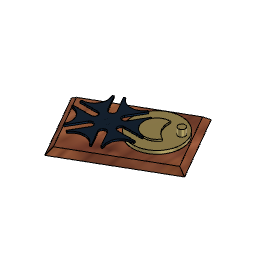
second mechanism v1 (Autodesk Fusion 360 design; units mm, degrees)
Autodesk Fusion 360 part; units mm, degrees
sketch "all" plane through (0, 0, 0) normal (0, 0, 1) x (1, 0, 0) in component "holder"
  circle A0 centre (-15, -0.013468) radius 19
  circle A1 centre (4, 10.956187) radius 7.95
  circle A2 centre (4, -0.013468) radius 2.099973
  line L0 (-15, -0.013468) -> (4, -0.013468) construction
  line L1 (4, -0.013468) -> (4, 10.956187) construction
  circle A3 centre (4, 10.956187) radius 10.969655 construction
  line L2 (4, 10.956187) -> (-5.5, 5.47136) construction
  line L3 (4, 2.086505) -> (-6.969655, 2.086505)
  arc A4 (-6.969655, 2.086505) -> (-6.969655, -2.113441) centre (-6.969655, -0.013468) ccw
  line L4 (-6.969655, -2.113441) -> (4, -2.113441)
  arc A5 (4, -2.113441) -> (4, 2.086505) centre (4, -0.013468) ccw
  line L5 (4, -0.013468) -> (-6.969655, -0.013468) construction
  circle A6 centre (-15, 21.925842) radius 7.95
  line L6 (-9.166198, 5.891028) -> (-3.68137, 15.391028)
  arc A7 (-12.803457, 7.991001) -> (-9.166198, 5.891028) centre (-10.984827, 6.941015) ccw
  line L7 (-7.31863, 17.491001) -> (-12.803457, 7.991001)
  arc A8 (-3.68137, 15.391028) -> (-7.31863, 17.491001) centre (-5.5, 16.441015) ccw
  circle A9 centre (-34, 10.956187) radius 7.95
  line L8 (-17.196543, 7.991001) -> (-22.68137, 17.491001)
  arc A10 (-20.833802, 5.891028) -> (-17.196543, 7.991001) centre (-19.015172, 6.941015) ccw
  line L9 (-26.31863, 15.391028) -> (-20.833802, 5.891028)
  arc A11 (-22.68137, 17.491001) -> (-26.31863, 15.391028) centre (-24.5, 16.441015) ccw
  circle A12 centre (-34, -10.983123) radius 7.95
  line L10 (-23.030345, 2.086505) -> (-34, 2.086505)
  arc A13 (-23.030345, -2.113441) -> (-23.030345, 2.086505) centre (-23.030345, -0.013468) ccw
  line L11 (-34, -2.113441) -> (-23.030345, -2.113441)
  arc A14 (-34, 2.086505) -> (-34, -2.113441) centre (-34, -0.013468) ccw
  circle A15 centre (-15, -21.952778) radius 7.95
  line L12 (-20.833802, -5.917964) -> (-26.31863, -15.417964)
  arc A16 (-17.196543, -8.017937) -> (-20.833802, -5.917964) centre (-19.015172, -6.967951) ccw
  line L13 (-22.68137, -17.517937) -> (-17.196543, -8.017937)
  arc A17 (-26.31863, -15.417964) -> (-22.68137, -17.517937) centre (-24.5, -16.467951) ccw
  circle A18 centre (4, -10.983123) radius 7.95
  line L14 (-12.803457, -8.017937) -> (-7.31863, -17.517937)
  arc A19 (-9.166198, -5.917964) -> (-12.803457, -8.017937) centre (-10.984827, -6.967951) ccw
  line L15 (-3.68137, -15.417964) -> (-9.166198, -5.917964)
  arc A20 (-7.31863, -17.517937) -> (-3.68137, -15.417964) centre (-5.5, -16.467951) ccw
  circle A21 centre (-15, -0.013468) radius 2
  line L16 (14.89621, 17.518771) -> (14.508328, 17.285157)
  line L17 (-34, -10.983123) -> (-45, 8.069436)
  line L18 (-34, -10.983123) -> (-23, -30.035682)
  line L19 (-45, 8.069436) -> (2.631397, 35.569436)
  line L20 (-23, -30.035682) -> (24.631397, -2.535682)
  line L21 (26.363448, -1.535682) -> (24.631397, -2.535682)
  line L22 (4.363448, 36.569436) -> (2.631397, 35.569436)
  circle A22 centre (4, 10.956187) radius 1.5
  circle A23 centre (4, 10.956187) radius 14.790733
  line L23 (30.693575, 0.964318) -> (8.693575, 39.069436)
  line L24 (30.693575, 0.964318) -> (26.363448, -1.535682)
  line L25 (8.693575, 39.069436) -> (4.363448, 36.569436)
  line L26 (4, 10.956187) -> (0.025, 17.841089)
  line L27 (4, 10.956187) -> (7.975, 4.071285)
  line L28 (-0.75, 8.213773) -> (22.60208, 21.696103)
  circle A24 centre (15.672989, 17.69559) radius 11.407497
  dimension "d3" = 38
  dimension "d8" = 360
  dimension "d9" = 4
  dimension "d10" = 15.9
  dimension "d11" = 22
  dimension "d12" = 22
  dimension "d13" = 55
  dimension "d14" = 55
  dimension "d15" = 55
  dimension "d17" = 3
  constraint horizontal L0
  constraint tangent A0 L1
  constraint perpendicular L0 L1
  constraint concentric A1 A3
  constraint tangent L3 A4
  constraint tangent A4 L4
  constraint parallel L3 L4
  constraint tangent L4 A5
  constraint tangent L3 A5
  constraint parallel L0 L5
  constraint equal A2 A5
  constraint equal L2 L5
  constraint concentric A0 A21
  constraint perpendicular L17 L19
  constraint perpendicular L18 L20
  constraint concentric A1 A22
  constraint concentric A3 A23
  constraint perpendicular L2 L26
  constraint perpendicular L2 L27
  constraint perpendicular L23 L28
  measures "d3" diameter of A0
  measures "d9" diameter of A21
  measures "d10" diameter of A1
  measures "d17" diameter of A22
extrude "Extrude1" add sketch "all" along normal blind 3 contours A0 A2 | A0 A2 A5 | A0 A2 L3 A4 L4 A23 | A0 A1 L3 A4 L6 A7 A23 | A0 A1 A2 L3 L4 A5 A18 A23 A24 | A0 L4 A18 A23 | A0 A1 | A0 A1 A22 L27 L28 | A0 A18 A23 | A0 A18 A23 | A0 A4 L4 A6 A7 L7 A9 L8 A10 L9 A12 L10 A13 L11 A15 L12 A16 L13 A18 L14 A19 L15 A23 | A4 L4 A23 | A0 A1 A22 L26 L28 | A0 A1 A6 L6 L7 A8 A23 A24 | A1 A22 L27 L28 A24 | A0 A18 L20 A23 | A0 A18 A23 | A18 L20 L21 A23 L23 L24 A24 | A22 L27 L28 | A22 L26 L28 | A0 L6 A7 L7 A23 | A0 L6 L7 A8 | A1 A22 L26 L28 A24 | A1 L28 A24 | A1 A23 L28 A24 | A22 L27 L28 | A7 L7 A23 | A0 A15 A18 L14 L15 A20 L20 | A23 L23 L28 A24 | A22 L26 L28 | A0 A6 L7 A23 | A1 A23 L28 A24 | A1 L28 A24 | A0 L14 L15 A20 | A0 L14 A19 L15 | A0 A6 A23 | A0 A6 A23 | A23 L23 L28 A24 | A6 L19 L22 A23 L23 L25 A24 | A0 A6 A23 | A0 A15 L20 | A0 A6 L19 A23 | A0 A6 A9 L8 L9 A11 L19 | A0 A15 | A0 A12 A15 L12 L13 A17 L18 L20 | A0 L8 A10 L9 | A0 L8 L9 A11 | A0 A9 L19 | A0 L12 L13 A17 | A0 L12 A16 L13 | A0 A12 L17 L18 | A0 A9 | A0 A9 A12 L10 L11 A14 L17 L19 | A0 A12 | A0 L10 A13 L11 | A0 L10 L11 A14 | A21 picked at (3.340785, -0.494) picked at (4.632432, -0.537651) picked at (-3.17387, 0.698163) picked at (-6.340252, 4.98624) picked at (12.935121, 4.420171) picked at (1.879299, -2.87092) picked at (-0.582937, 9.637776) picked at (5.326479, 6.328407) picked at (4.404901, -3.398007) picked at (3.109319, -3.488085) picked at (-15, -10.012884) picked at (-6.003482, -0.913731) picked at (0.655464, 14.418841) picked at (2.807204, 21.962237) picked at (7.105875, 7.493261) picked at (3.845681, -12.704019) picked at (-0.187956, -8.954474) picked at (16.605485, -3.4837) picked at (3.364932, 10.187032) picked at (3.102803, 10.520356) picked at (-7.870935, 10.188718) picked at (-5.200601, 17.064211) picked at (2.553956, 15.377417) picked at (7.908869, 12.26239) picked at (15.28476, 8.588295) picked at (4.863604, 10.457585) picked at (-11.281391, 8.227876) picked at (-4.105681, -18.778361) picked at (20.961309, 15.264678) picked at (3.564169, 11.853384) picked at (-9.034977, 16.03316) picked at (7.467298, 21.954992) picked at (7.064846, 13.715008) picked at (-5.200601, -17.091146) picked at (-8.956272, -10.014003) picked at (-8.954447, 17.40697) picked at (-8.228646, 18.483939) picked at (16.164617, 23.537533) picked at (-2.213683, 29.107518) picked at (-15.337117, 17.284641) picked at (-13.539598, -22.688302) picked at (-16.567499, 22.652646) picked at (-25.894319, 18.751425) picked at (-15, -17.309725) picked at (-25.186526, -24.130917) picked at (-20.638853, 10.220822) picked at (-24.799399, 17.064211) picked at (-33.906781, 12.588695) picked at (-24.799399, -17.091146) picked at (-21.043728, -10.014003) picked at (-35.032086, -6.9354) picked at (-30.028913, 8.551739) picked at (-40.979586, 3.223467) picked at (-30.028913, -8.578675) picked at (-26.682581, -0.247223) picked at (-34.689403, 0.038842) picked at (-14.399354, -0.302724) makes body 1 in component "holder"
extrude "Extrude2" add sketch "all" along normal blind 6 and the other way blind -4 separate body contours A0 A2 | A0 A2 A5 | A0 A2 L3 A4 L4 A23 | A0 A1 L3 A4 L6 A7 A23 | A0 A1 A2 L3 L4 A5 A18 A23 A24 | A0 L4 A18 A23 | A0 A1 | A0 A1 A22 L27 L28 | A0 A18 A23 | A0 A18 A23 | A0 A1 A22 L26 L28 | A0 A1 A6 L6 L7 A8 A23 A24 | A1 A22 L27 L28 A24 | A22 L27 L28 | A22 L26 L28 | A0 L6 A7 L7 A23 | A0 L6 L7 A8 | A1 A22 L26 L28 A24 | A1 L28 A24 | A1 A23 L28 A24 | A22 L27 L28 | A22 L26 L28 | A0 A6 L7 A23 | A1 A23 L28 A24 | A1 L28 A24 | A0 A6 A23 | A0 A6 A23 picked at (3.340785, -0.494) picked at (4.632432, -0.537651) picked at (-3.17387, 0.698163) picked at (-6.340252, 4.98624) picked at (12.935121, 4.420171) picked at (1.879299, -2.87092) picked at (-0.582937, 9.637776) picked at (5.326479, 6.328407) picked at (4.404901, -3.398007) picked at (3.109319, -3.488085) picked at (0.655464, 14.418841) picked at (2.807204, 21.962237) picked at (7.105875, 7.493261) picked at (3.364932, 10.187032) picked at (3.102803, 10.520356) picked at (-7.870935, 10.188718) picked at (-5.200601, 17.064211) picked at (2.553956, 15.377417) picked at (7.908869, 12.26239) picked at (15.28476, 8.588295) picked at (4.863604, 10.457585) picked at (3.564169, 11.853384) picked at (-9.034977, 16.03316) picked at (7.467298, 21.954992) picked at (7.064846, 13.715008) picked at (-8.954447, 17.40697) picked at (-8.228646, 18.483939) makes body 2 in component "holder"
extrude "Extrude3" add sketch "all" along normal blind 6 and the other way blind -7 contours A0 A1 | A0 A1 A22 L27 L28 | A0 A1 A22 L26 L28 | A1 A22 L27 L28 A24 | A22 L27 L28 | A22 L26 L28 | A1 A22 L26 L28 A24 | A1 L28 A24 | A22 L27 L28 | A22 L26 L28 | A1 L28 A24 picked at (0.566754, 7.646453) picked at (5.326479, 6.328407) picked at (0.655464, 14.418841) picked at (7.105875, 7.493261) picked at (4.435831, 10.058991) picked at (3.102803, 10.520356) picked at (2.553956, 15.377417) picked at (7.908869, 12.26239) picked at (4.863604, 10.457585) picked at (3.564169, 11.853384) picked at (7.064846, 13.715008) bodies 2 in component "holder"
extrude "Extrude4" add sketch "all" along normal blind 10 and the other way blind -6 contours A0 A2 | A0 A2 L3 L4 A5 picked at (3.340776, 0.467237) picked at (4.632426, 0.510894) bodies 2 in component "holder"
copy_body "CutPasteBodies1" bodies 2 removing the originals makes body 3 in component "crank"
extrude "Extrude5" add sketch "all" along normal blind 7 and the other way blind -6 separate body contours A0 A1 L3 A4 L6 A7 A23 | A0 L4 A18 A23 | A0 A4 L4 A6 A7 L7 A9 L8 A10 L9 A12 L10 A13 L11 A15 L12 A16 L13 A18 L14 A19 L15 A23 | A0 A6 L7 A23 | A21 picked at (-6.340252, 4.98624) picked at (1.879358, -2.870385) picked at (-15, -10.012884) picked at (-9.034977, 16.03316) picked at (-14.399354, -0.302724) makes body 4 in component "holder"
copy_body "CutPasteBodies1'" bodies 4 body 4 seen with x (0.5, 0.8660254, 0) y (-0.8660254, 0.5, 0) z (0, 0, 1) at (-7.511664, 12.983647, 0) removing the originals makes body 5 in component "snowflake"
extrude "Extrude6" add sketch "all" along normal blind 6.5 contours A21 picked at (-14.399354, -0.302724) bodies 1 in component "holder"
extrude "Extrude7" add sketch "all" along normal blind 5 contours A22 L27 L28 | A22 L26 L28 | A22 L27 L28 | A22 L26 L28 picked at (4.435831, 10.058991) picked at (3.102803, 10.520356) picked at (4.863604, 10.457585) picked at (3.564169, 11.853384) bodies 1 in component "holder"
chamfer "Chamfer1" distance 3 angle 45 4 edges at (3.846788, -14.535682, 3) (19.693575, 20.016877, 3) (-18.153212, 23.569436, 3) (-34, -10.983123, 3) on bodies 1 in component "holder"
extrude "Extrude1'" cut sketch "all" along normal blind 7 and the other way blind -6 contours A0 A1 | A0 A1 A22 L27 L28 | A0 A1 A22 L26 L28 | A1 A22 L27 L28 A24 | A22 L27 L28 | A22 L26 L28 | A1 A22 L26 L28 A24 | A1 L28 A24 | A22 L27 L28 | A22 L26 L28 | A1 L28 A24 picked at (0.566754, 7.646453) picked at (5.326479, 6.328407) picked at (0.655464, 14.418841) picked at (7.105875, 7.493261) picked at (4.435831, 10.058991) picked at (3.102803, 10.520356) picked at (2.553956, 15.377417) picked at (7.908869, 12.26239) picked at (4.863604, 10.457585) picked at (3.564169, 11.853384) picked at (7.064846, 13.715008) sketch seen with x (-0.5, -0.8660254, 0) y (0.8660254, -0.5, 0) z (0, 0, 1) at (-3.488336, 19.898382, 0) bodies 3 in component "crank"
extrude "Extrude8" add sketch "all" along normal blind 7 and the other way blind -6 separate body contours A0 A1 | A0 A1 A22 L27 L28 | A0 A1 A22 L26 L28 | A1 A22 L27 L28 A24 | A22 L27 L28 | A22 L26 L28 | A1 A22 L26 L28 A24 | A22 L27 L28 | A22 L26 L28 picked at (0.566754, 7.646453) picked at (5.326479, 6.328407) picked at (0.655464, 14.418841) picked at (7.105875, 7.493261) picked at (4.435831, 10.058991) picked at (3.102803, 10.520356) picked at (2.553956, 15.377417) picked at (4.863604, 10.457585) picked at (3.564169, 11.853384) makes body 6 in component "holder"
copy_body "CutPasteBodies2" bodies 6 body 6 seen with x (-0.5, -0.8660254, 0) y (0.8660254, -0.5, 0) z (0, 0, 1) at (-3.488336, 19.898382, 0) removing the originals makes body 7 in component "crank"
combine "Combine1" operation add target body 7 tool bodies 3 in component "crank"
component "holder" placed x (1, 0, 0) y (0, 1, 0) z (0, 0, 1) at (0, 0, 0)
component "crank" placed x (-0.5, 0.8660254, 0) y (-0.8660254, -0.5, 0) z (0, 0, 1) at (15.488337, 12.970179, 0)
component "snowflake" placed x (-0.99999999, 0.00013915, 0) y (-0.00013915, -0.99999999, 0) z (0, 0, 1) at (-30.000002, -0.024849, 0)
named bodies: "holder", "crank", "snowflake", "crank2"
